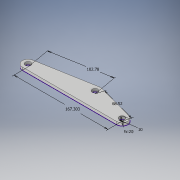
# Autodesk Inventor part: test3
Saved by Autodesk Inventor 2019 (Build 230136000, 136)
## iProperties
Created: 2021-02-18
Part Number: test3
Material: 一般
Document SubType Name: Modeling
Designer: wasd5
Density: 1 g/cm^3
Appearance: 預設
Author: wasd5
Autodesk Inventor part; units mm, degrees
ref_plane "YZ Plane" through (0, 0, 0) normal (1, 0, 0) x (0, 1, 0)
ref_plane "XZ Plane" through (0, 0, 0) normal (0, 1, 0) x (-1, 0, 0)
ref_plane "XY Plane" through (0, 0, 0) normal (0, 0, 1) x (1, 0, 0)
sketch "草圖2" plane through (0, 0, 0) normal (0, 1, 0) x (-1, 0, 0)
  line L0 (-101.1907, -18.0045) -> (0, 0) construction
  line L1 (0, 0) -> (-167.303, 0) construction
  arc A0 (-167.303, 10) -> (-169.9306, -9.6486) centre (-167.303, 0) ccw
  arc A1 (1.7517, -9.8454) -> (0, 10) centre (0, 0) ccw
  line L2 (-167.303, 10) -> (0, 10)
  line L3 (-169.9306, -9.6486) -> (-103.8184, -27.6531)
  line L4 (-167.303, 0) -> (-101.1907, -18.0045) construction
  arc A2 (-103.8184, -27.6531) -> (-99.439, -27.8498) centre (-101.1907, -18.0045) ccw
  line L5 (1.7517, -9.8454) -> (-99.439, -27.8498)
  circle A3 centre (-167.303, 0) radius 5
  circle A4 centre (0, 0) radius 5
  circle A5 centre (-101.1907, -18.0045) radius 5
  dimension "d11" = 20
  dimension "hole" = 10
  dimension "center_distance1" = 167.303
  dimension "center_distance3" = 68.52
  dimension "center_distance2" = 102.78
  constraints: 12 end point, 7 coincident, 6 centre point, 6 point on circle, 6 tangent, 4 equal radius, 1 horizontal
  measures "d11" diameter of A0
  measures "hole" diameter of A3
  measures "center_distance1" distance of L1.start L1.end
  measures "center_distance3" distance of L4.start L4.end
  measures "center_distance2" distance of L4.end L1.start
extrude "擠出2" add sketch "草圖2" along normal blind 5
equation "\"d11\" = 2 * hole"
